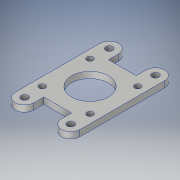
# Autodesk Inventor part: Piston Motor holder
Saved by Autodesk Inventor 2018.1 (Build 221171000, 171)
## iProperties
Created: 2013-10-18
Part Number: Piston Motor holder
Material: Aluminum 6061
Document SubType Name: Modeling
Designer: Gabriel Smolnycki
Mass: 18.748 g
Surface Area: 51.9029 cm^2
Volume: 6.94369 cm^3
Density: 2.7 g/cm^3
Appearance: Aluminum - Flat
Author: Gabriel Smolnycki
Sending System: SolidWorks 2017
Last Author: Gabriel Smolnycki
Last Saved: 2017-09-14
Autodesk Inventor part; units mm, degrees
ref_plane "YZ Plane" through (0, 0, 0) normal (1, 0, 0) x (0, 1, 0)
ref_plane "XZ Plane" through (0, 0, 0) normal (0, 1, 0) x (-1, 0, 0)
ref_plane "XY Plane" through (0, 0, 0) normal (0, 0, 1) x (1, 0, 0)
sketch "Sketch1" plane through (0, 0, 0) normal (0, 1, 0) x (-1, 0, 0)
  arc A0 (9, -27.5) -> (21, -27.5) centre (15, -27.5) ccw
  arc A1 (-9, 27.5) -> (-21, 27.5) centre (-15, 27.5) ccw
  arc A2 (21, 27.5) -> (9, 27.5) centre (15, 27.5) ccw
  arc A3 (-21, -27.5) -> (-9, -27.5) centre (-15, -27.5) ccw
  line L0 (-9, 21) -> (-9, 27.5)
  line L1 (-9, -21) -> (9, -21)
  circle A4 centre (0, 0) radius 12
  line L2 (21, -27.5) -> (21, 27.5)
  line L3 (-21, 27.5) -> (-21, -27.5)
  line L4 (9, 21) -> (-9, 21)
  line L5 (9, -21) -> (9, -27.5)
  line L6 (-9, -27.5) -> (-9, -21)
  line L7 (9, 27.5) -> (9, 21)
  constraints: 16 end point, 8 point on circle, 6 vertical, 5 centre point, 5 equal length, 3 equal radius, 2 horizontal, 1 collinear
extrude "Extrusion1" add sketch "Sketch1" against normal blind 4.064
hole "Hole8" at (-15.5, -4.064, -15.5) direction (0, 1, 0) diameter 4 depth 4.064
hole "Hole7" at (-15.5, -4.064, 15.5) direction (0, 1, 0) diameter 4 depth 4.064
hole "Hole6" at (15.5, -4.064, 15.5) direction (0, 1, 0) diameter 4 depth 4.064
hole "Hole5" at (15.5, -4.064, -15.5) direction (0, 1, 0) diameter 4 depth 4.064
sketch "Sketch5" plane through (0, -4.064, 0) normal (0, -1, 0) x (1, 0, 0)
  point P0 (15.5, -15.5)
hole "Hole4" at (15, -4.064, -27.5) direction (0, 1, 0) diameter 4.5 depth 4.064
sketch "Sketch4" plane through (0, -4.064, 0) normal (0, -1, 0) x (1, 0, 0)
  point P0 (15.5, 15.5)
hole "Hole3" at (15, -4.064, 27.5) direction (0, 1, 0) diameter 4.5 depth 4.064
sketch "Sketch3" plane through (0, -4.064, 0) normal (0, -1, 0) x (1, 0, 0)
  point P0 (-15.5, 15.5)
hole "Hole2" at (-15, -4.064, 27.5) direction (0, 1, 0) diameter 4.5 depth 4.064
sketch "Sketch2" plane through (0, -4.064, 0) normal (0, -1, 0) x (1, 0, 0)
  point P0 (-15.5, -15.5)
hole "Hole1" at (-15, -4.064, -27.5) direction (0, 1, 0) diameter 4.5 depth 4.064
sketch "Sketch6" plane through (0, -4.064, 0) normal (0, -1, 0) x (1, 0, 0)
  point P0 (15, -27.5)
sketch "Sketch7" plane through (0, -4.064, 0) normal (0, -1, 0) x (1, 0, 0)
  point P0 (15, 27.5)
sketch "Sketch8" plane through (0, -4.064, 0) normal (0, -1, 0) x (1, 0, 0)
  point P0 (-15, 27.5)
sketch "Sketch9" plane through (0, -4.064, 0) normal (0, -1, 0) x (1, 0, 0)
  point P0 (-15, -27.5)
body "Solid3"
